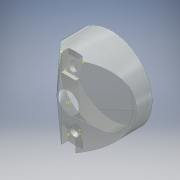
# Autodesk Inventor part: LightShieldBottom
Saved by Autodesk Inventor 2016 (Build 200138000, 138)
## iProperties
Created: 2015-11-30
Part Number: LightShieldBottom
Material: Glass
Document SubType Name: Modeling
Designer: Vervaeke-Lab
Density: 2.18 g/cm^3
Appearance: Clear
Mass: 13.5613 g
Surface Area: 51.4091 cm^2
Volume: 6.22076 cm^3
Author: Vervaeke-Lab
Autodesk Inventor part; units mm, degrees
ref_plane "YZ Plane" through (0, 0, 0) normal (1, 0, 0) x (0, 1, 0)
sketch "Sketch1" plane through (0, 0, 0) normal (0, 1, 0) x (-1, 0, 0)
  circle A0 centre (0, 0) radius 19
  dimension "d0" = 38
  constraints: 1 centre point, 1 coincident
  measures "d0" diameter of A0
extrude "Extrusion1" add sketch "Sketch1" along normal blind 20
sketch "Sketch2" plane through (0, 0, 0) normal (0, -1, 0) x (1, 0, 0)
  line L0 (0, -10.5) -> (3.4, -10.5)
  line L1 (3.4, -10.5) -> (3.4, -19)
  line L2 (3.4, -19) -> (0, -19)
  line L3 (0, -19) -> (-3.4, -19)
  line L4 (-3.4, -19) -> (-3.4, -10.5)
  line L5 (-3.4, -10.5) -> (0, -10.5)
  point P0 (0, 0)
  dimension "d3" = 10.5
  dimension "d5" = 8.5
  dimension "d113" = 3.4
  dimension "d114" = 3.4
  constraints: 12 end point, 4 perpendicular, 2 point on line, 1 horizontal
  measures "d3" distance of point (0, 0) L0.start
  measures "d5" distance of L0.end L1.end
  measures "d113" distance from line of point (0, 0) L1
  measures "d114" distance from line of point (0, 0) L4
sketch "Sketch3" plane through (0, 0, 0) normal (0, -1, 0) x (1, 0, 0)
  line L0 (0.251, 10.5) -> (3.4, 10.5)
  line L1 (3.4, 10.5) -> (3.4, 19)
  line L2 (3.4, 19) -> (-0.351, 19)
  line L3 (-0.351, 19) -> (-3.4, 19)
  line L4 (-3.4, 19) -> (-3.4, 10.5)
  line L5 (-3.4, 10.5) -> (0.251, 10.5)
  point P0 (0, 0)
  dimension "d22" = 8.5
  dimension "d106" = 10.5
  dimension "d107" = 3.4
  dimension "d110" = 3.4
  constraints: 12 end point, 2 point on line, 1 other
  measures "d22" distance of L0.end L1.end
  measures "d106" distance from line of point (0, 0) L5
  measures "d107" distance from line of point (0, 0) L4
  measures "d110" distance from line of point (0, 0) L1
extrude "Extrusion2" cut sketch "Sketch3" against normal blind 3.22
extrude "Extrusion3" cut sketch "Sketch2" against normal blind 3.22
sketch "Sketch4" plane through (0, 0, 0) normal (1, 0, 0) x (0, 1, 0)
  line L0 (0, -10.5) -> (3.22, -10.5) projected
  line L1 (3.22, -10.5) -> (3.22, -16.6)
  line L2 (3.22, -10.5) -> (3.22, -18.6933) projected
  line L3 (3.22, -16.6) -> (3.22, -10.5)
  line L4 (3.22, -10.5) -> (1.52, -10.5)
  line L5 (1.52, -10.5) -> (3.22, -16.6)
  line L6 (-0.644, 0) -> (3.864, 0) projected
  point P0 (0, 0)
  dimension "d28" = 6.1
  dimension "d29" = 1.7
  constraints: 8 end point, 2 point on line, 1 collinear
  measures "d28" distance of L0.end L1.end
  measures "d29" distance of L0.end L4.end
revolve "Revolution1" add sketch "Sketch4" angle 360 about axis through (0, -10, 0) along (0, 1, 0)
sketch "Sketch5" plane through (0, 20, 0) normal (0, 1, 0) x (1, 0, 0)
  circle A0 centre (0, 0) radius 4.81
  dimension "d31" = 9.62
  constraints: 1 centre point, 1 coincident
  measures "d31" diameter of A0
extrude "Extrusion4" cut sketch "Sketch5" against normal through all
sketch "Sketch6" plane through (0, 0, 0) normal (1, 0, 0) x (0, 1, 0)
  line L0 (0, -4.81) -> (13.0829, -17.01)
  line L1 (20, -19) -> (20, 19) projected
  line L2 (13.0829, -4.81) -> (0, -4.81)
  line L3 (-2.6166, 0) -> (15.6995, 0) projected
  line L4 (13.0829, -4.81) -> (13.0829, -17.01)
  line L5 (3.22, -19) -> (20, -19) projected
  line L6 (0, -4.81) -> (13.0829, -4.81) construction
  point P0 (0, 0)
  point P1 (20, -4.81)
  point P2 (13.0829, -17.01)
  dimension "d85" = 12.2
  dimension "d90" = 13.0829
  constraints: 8 end point, 2 point on line, 1 coincident, 1 horizontal, 1 perpendicular
  measures "d85" distance of L0.end L2.start
  measures "d90" distance of L2.start L0.start
revolve "Revolution2" cut sketch "Sketch6" angle 360 about axis through (0, -10, 0) along (0, 1, 0)
ref_plane "Work Plane1" through (3.4, 3.22, 16.2481) normal (0, -0.9654954, 0.2604203) x (-0.7523847, -0.1715451, -0.6359949)
sketch "Sketch10" plane through (3.4, 3.22, 16.2481) normal (0, -0.9654954, 0.2604203) x (-0.7523847, -0.1715451, -0.6359949)
  line L0 (9.3243, 0.3271) -> (9.0379, 0) projected
  line L1 (-1.5552, -1.7763) -> (0, 0) projected
  line L2 (9.0379, 0) -> (0, 0)
  circle A0 centre (4.519, 0) radius 2
  point P0 (13.4442, 10.1942)
  dimension "d111" = 4
  constraints: 2 end point, 1 centre point, 1 horizontal, 1 midpoint
  measures "d111" diameter of A0
extrude "Extrusion5" cut sketch "Sketch10" along normal mid plane 4
ref_plane "Work Plane4" through (3.4, 1.6696, -10.5) normal (0, -0.9654954, -0.2604203) x (-0.7523847, 0.1715451, -0.6359949)
sketch "Sketch12" plane through (3.4, 1.6696, -10.5) normal (0, -0.9654954, -0.2604203) x (-0.7523847, 0.1715451, -0.6359949)
  line L0 (-0.2864, -0.3271) -> (0, 0) projected
  ellipse E0 centre (-3.8539, -9.5633) end of major axis (8.6357, -20.4981) minor radius 16.0272 (9.0379, 0) -> (3.9217, 4.4793) ccw projected
  line L1 (0, 0) -> (3.9217, 4.4793)
  line L2 (4.8298, -4.8065) -> (5.1162, -4.4793) projected
  line L3 (5.1162, -4.4793) -> (3.9217, 4.4793)
  line L4 (10.5931, 1.7763) -> (9.0379, 0) projected
  line L5 (9.0379, 0) -> (0, 0)
  circle A0 centre (4.519, 0) radius 2
  point P0 (-4.4062, -10.1942)
  point P1 (4.519, 0)
  dimension "d116" = 4
  constraints: 6 end point, 4 midpoint, 1 centre point, 1 coincident, 1 horizontal, 4 other
  measures "d116" diameter of A0
extrude "Extrusion6" cut sketch "Sketch12" along normal mid plane 4 contours A0 L3 L5 | L5 L3 A0 | L3 L5 A0 | L3 A0 L5
sketch "Sketch18" plane through (0, 0, 0) normal (0.1099078, 0, 0.9939418) x (0.9939418, 0, -0.1099078)
  line L0 (19, 20) -> (-19, 20) projected
  line L1 (19, 0) -> (5.4339, 0)
  line L2 (4.5334, 0) -> (5.4339, 0) projected
  line L3 (5.4339, 0) -> (19, 12.6506)
  line L4 (19, 0) -> (19, 20) projected
  line L5 (5.4339, 0) -> (23.9832, 0) construction
  line L6 (1.3249, 0) -> (19, 0) projected
  line L7 (19, 12.6506) -> (19, 0)
  line L8 (19, 0) -> (19, 20) projected
  line L9 (19, 0) -> (5.4339, 0)
  point P0 (0, 0)
  point P1 (24.4257, 20)
  dimension "d91" = 43
  constraints: 10 end point, 2 collinear, 2 point on line, 1 equal length, 1 horizontal
  measures "d91" angle of L5 L3
sketch "Sketch20" plane through (0, 0, 0) normal (-0.1099078, 0, 0.9939418) x (0.9939418, 0, 0.1099078)
  line L0 (5.4339, 3.22) -> (5.4339, 0) projected
  line L1 (5.4339, 0) -> (19, 12.6506)
  line L2 (19, 0) -> (19, 20) projected
  line L3 (5.4339, 0) -> (23.9832, 0) construction
  line L4 (1.3249, 0) -> (19, 0) projected
  line L5 (19, 12.6506) -> (19, 0)
  line L6 (5.4339, 0) -> (4.5334, 0) projected
  line L7 (19, 0) -> (5.4339, 0)
  point P0 (0, 0)
  point P1 (10.438, 5)
  point P2 (-18.8849, 20)
  point P3 (-18.8849, 20)
  dimension "d94" = 43
  constraints: 8 end point, 2 perpendicular, 1 equal length, 1 horizontal, 1 point on line, 2 other
  measures "d94" angle of L3 L1
sketch "Sketch21" plane through (0, 0, 0) normal (-0.1099078, 0, 0.9939418) x (0.9939418, 0, 0.1099078)
  point P0 (0, 0)
sketch "Sketch22" plane through (0, 0, 0) normal (-0.1099078, 0, 0.9939418) x (0.9939418, 0, 0.1099078)
  line L0 (-18.8849, 20) -> (-19, 20) projected
  line L1 (-5.4339, 0) -> (21.9126, 0) construction
  line L2 (-5.4339, 0) -> (-4.5334, 0) projected
  line L3 (-5.4339, 0) -> (-19, 14.5478)
  line L4 (-19, 0) -> (-19, 20) projected
  line L5 (-5.4339, 0) -> (14.4577, 0) construction
  line L6 (-19, 0) -> (-1.3249, 0) projected
  line L7 (-19, 14.5478) -> (-19, 0)
  line L8 (-19, 0) -> (-5.4339, 0)
  point P0 (0, 0)
  dimension "d97" = 133
  constraints: 10 end point, 2 horizontal, 2 perpendicular, 1 equal length, 1 point on line
  measures "d97" angle of L5 L3
sketch "Sketch23" plane through (0, 0, 0) normal (0.1099078, 0, 0.9939418) x (0.9939418, 0, -0.1099078)
  line L0 (-9.5907, 0) -> (-1.3249, 0) projected
  line L1 (-5.6359, 0) -> (1.2007, 0) construction
  line L2 (-4.5334, 0) -> (-5.4339, 0) projected
  line L3 (-5.4339, 0) -> (-19, 14.5478)
  line L4 (-19, 0) -> (-19, 20) projected
  line L5 (-5.4339, 0) -> (14.4577, 0) construction
  line L6 (-19, 0) -> (-1.3249, 0) projected
  line L7 (-19, 14.5478) -> (-19, 0)
  line L8 (-19, 0) -> (-5.4339, 0)
  point P0 (0, 0)
  point P1 (-18.8849, 20)
  point P2 (-18.8849, 20)
  dimension "d100" = 133
  constraints: 10 end point, 2 horizontal, 2 point on line, 1 coincident, 1 collinear, 1 equal length, 1 perpendicular
  measures "d100" angle of L5 L3
extrude "Extrusion13" cut sketch "Sketch18" along normal through all both and the other way through all
extrude "Extrusion14" cut sketch "Sketch20" along normal through all both and the other way through all
extrude "Extrusion15" cut sketch "Sketch22" along normal through all both and the other way through all
extrude "Extrusion16" cut sketch "Sketch23" along normal through all both and the other way through all
sketch "Sketch25" plane through (0, 20, 0) normal (0, 1, 0) x (1, 0, 0)
  circle A0 centre (0, 0) radius 17
  dimension "d103" = 34
  constraints: 1 centre point, 1 coincident
  measures "d103" diameter of A0
extrude "Extrusion17" cut sketch "Sketch25" against normal blind 6.92
body "Solid1"
